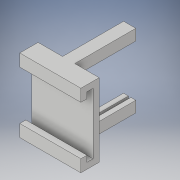
# Autodesk Inventor part: Substrategrip90degreesThick
Saved by Autodesk Inventor 2019 (Build 230136000, 136)
## iProperties
Created: 2018-09-07
Part Number: Substrategrip90degreesThick
Material: Generic
Document SubType Name: Modeling
Designer: s152529
Density: 1 g/cm^3
Appearance: Default
Author: s152529
Autodesk Inventor part; units mm, degrees
ref_plane "YZ Plane" through (0, 0, 0) normal (1, 0, 0) x (0, 1, 0)
ref_plane "XZ Plane" through (0, 0, 0) normal (0, 1, 0) x (-1, 0, 0)
ref_plane "XY Plane" through (0, 0, 0) normal (0, 0, 1) x (1, 0, 0)
sketch "Sketch1" plane through (0, 0, 0) normal (0, 0, 1) x (1, 0, 0)
  line L0 (-25, 30) -> (25, 30)
  line L1 (25, 30) -> (25, -30)
  line L2 (25, -30) -> (-25, -30)
  line L3 (-25, -30) -> (-25, 30)
  point P0 (0, 0)
  dimension "d0" = 50
  dimension "d1" = 60
  dimension "d2" = 30
  dimension "d3" = 25
  constraints: 8 end point, 2 parallel, 1 horizontal, 1 perpendicular
  measures "d0" distance of L1.end L2.end
  measures "d1" distance between parallel lines of L2 L0
  measures "d2" distance from line of L0 point (0, 0)
  measures "d3" distance from line of point (0, 0) L3
extrude "Extrusion1" add sketch "Sketch1" along normal blind 5
sketch "Sketch2" plane through (0, 0, 5) normal (0, 0, 1) x (1, 0, 0)
  line L0 (-25, 30) -> (-25, -30) projected
  line L1 (-25, 25) -> (25, 25)
  line L2 (25, -30) -> (25, 30) projected
  line L3 (25, 30) -> (-25, 30) projected
  point P0 (0, 0)
  dimension "d6" = 5
  constraints: 2 end point, 2 point on line, 1 horizontal
  measures "d6" distance between parallel lines of L3 L1
extrude "Extrusion2" add sketch "Sketch2" along normal blind 10
sketch "Sketch3" plane through (0, 0, 5) normal (0, 0, 1) x (1, 0, 0)
  line L0 (-25, -30) -> (-25, 30) projected
  line L1 (-25, -25) -> (25, -25)
  line L2 (25, 30) -> (25, -30) projected
  line L3 (-25, -30) -> (25, -30) projected
  point P0 (0, 0)
  dimension "d9" = 5
  constraints: 2 end point, 2 point on line, 1 horizontal
  measures "d9" distance between parallel lines of L3 L1
extrude "Extrusion3" add sketch "Sketch3" along normal blind 10
sketch "Sketch4" plane through (-25, -25, 5) normal (0, 1, 0) x (1, 0, 0)
  line L0 (0, 5) -> (0, -10) projected
  line L1 (0, -5) -> (50, -5)
  line L2 (50, 5) -> (50, -10) projected
  line L3 (0, -10) -> (50, -10) projected
  point P0 (25, 5)
  dimension "d12" = 5
  constraints: 2 end point, 2 point on line, 1 horizontal
  measures "d12" distance between parallel lines of L3 L1
extrude "Extrusion4" add sketch "Sketch4" along normal blind 5
sketch "Sketch5" plane through (-25, 25, 5) normal (0, -1, 0) x (1, 0, 0)
  line L0 (0, -5) -> (0, 10) projected
  line L1 (0, 5) -> (50, 5)
  line L2 (50, -5) -> (50, 10) projected
  line L3 (50, 10) -> (0, 10) projected
  point P0 (25, -5)
  dimension "d15" = 5
  constraints: 2 end point, 2 point on line, 1 horizontal
  measures "d15" distance between parallel lines of L3 L1
extrude "Extrusion5" add sketch "Sketch5" along normal blind 5
sketch "Sketch12" plane through (0, 0, 0) normal (0, 0, -1) x (-1, 0, 0)
  line L0 (25, 30) -> (-25, 30) projected
  line L1 (-5, 30) -> (5, 30)
  line L2 (5, 30) -> (5, 25)
  line L3 (5, 25) -> (-5, 25)
  line L4 (-5, 25) -> (-5, 30)
  line L5 (-25, 30) -> (-25, -30) projected
  line L6 (-5, 25) -> (-1, 25)
  line L7 (-1, 25) -> (-1, 21)
  line L8 (-1, 21) -> (-5, 21)
  line L9 (-5, 21) -> (-5, 25)
  line L10 (5, 25) -> (1, 25)
  line L11 (1, 25) -> (1, 21)
  line L12 (1, 21) -> (5, 21)
  line L13 (5, 21) -> (5, 25)
  point P0 (0, 0)
  dimension "d42" = 10
  dimension "d43" = 5
  dimension "d44" = 20
  dimension "d45" = 4
  dimension "d46" = 4
  dimension "d47" = 4
  dimension "d50" = 4
  constraints: 24 end point, 6 parallel, 3 horizontal, 3 perpendicular, 1 point on line
  measures "d42" distance of L2.end L3.end
  measures "d43" distance of L1.end L2.end
  measures "d44" distance between parallel lines of L5 L4
  measures "d45" distance of L7.end L8.end
  measures "d46" distance of L6.end L7.end
  measures "d47" distance of L12.end L11.end
  measures "d50" distance between parallel lines of L10 L12
extrude "Extrusion12" add sketch "Sketch12" along normal blind 50
mirror "Mirror1" about plane through (0, 0, 0) normal (0, 1, 0) of "Extrusion12"
body "Solid1"
